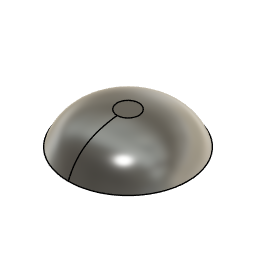
hub (Autodesk Fusion 360 archive; units mm, degrees)
design "daszek2"
Autodesk Fusion 360 part; units mm, degrees
sketch "Sketch1" plane through (0, 0, 0) normal (1, 0, 0) x (0, 1, 0)
  spline S0 degree 5 poles (-20, 0) (-22.7257, -0.3253) (-28.0984, -1.0502) (-35.9212, -2.3607) (-45.8716, -4.5618) (-57.453, -8.1224) (-68.0948, -12.571) (-77.709, -17.9907) (-86.2289, -24.4443) (-93.6692, -31.9182) (-100.0996, -40.3463) (-104.4963, -47.7952) (-107.3992, -53.7549) (-109.1618, -57.8911) (-110, -60) knots 0 0 0 0 0 0 0.1 0.2 0.3 0.4 0.5 0.6 0.7 0.8 0.9 1 1 1 1 1 1
  spline S1 degree 3 poles (-19.6445, -2.9789) (-34.008, -4.693) (-47.0407, -7.6194) (-58.39, -11.9827) (-67.6436, -15.5402) (-75.7205, -20.0828) (-82.5658, -25.7517) (-91.5958, -33.2299) (-98.5876, -42.6658) (-103.9793, -53.7643) (-105.1319, -56.1368) (-106.2094, -58.5851) (-107.2121, -61.108) knots 0 0 0 0 0.320426 0.320426 0.320426 0.581685 0.581685 0.581685 0.926327 0.926327 0.926327 1 1 1 1
  line L0 (0, 0) -> (0, -2.9702)
  line L1 (-110, -60) -> (-106.765, -60)
  line L2 (-20, 0) -> (0, 0)
  line L3 (-19.6445, -2.9789) -> (0, -2.9702)
  point P0 (-80, -20)
  dimension "d1" = 110
  dimension "d2" = 60
  dimension "d3" = 80
  dimension "d4" = 20
  dimension "d5" = -3
  dimension "d18" = 20
  constraint vertical L0
  constraint coincident S1 L1.end
  constraint perpendicular L0 L1
  constraint coincident L0.start L2.end
  constraint perpendicular L0 L2
  measures "d1" distance of L0.start S0.end
  measures "d2" distance of L0.start S0.end
  measures "d3" horizontal distance of L0.start P0
  measures "d4" vertical distance of L0.start P0
  measures "d18" distance of L0.start S0.start
revolve "Revolve1" add sketch "Sketch1" angle 360 about axis through (0, 0, 1.75) along (0, 0, 1)
ref_plane "WorkPlane1" through (0, 0, -2) normal (0, 0, 1) x (1, 0, 0)
sketch "Sketch2" plane through (0, 0, -2) normal (0, 0, 1) x (1, 0, 0)
  circle A0 centre (0, 0) radius 22.5
  dimension "d7" = 45
  constraint coincident A0.centre origin
  measures "d7" diameter of A0
extrude "Extrude1" add sketch "Sketch2" against normal blind 25
sketch "Sketch3" plane through (0, 0, -27) normal (0, 0, -1) x (1, 0, 0)
  circle A0 centre (0, 0) radius 22.5
  circle A1 centre (10.6066, -10.6066) radius 2.05
  circle A2 centre (3.8823, 14.4889) radius 2.05
  circle A3 centre (-14.4889, -3.8823) radius 2.05
  line L0 (0, 0) -> (10.6066, -10.6066) construction
  dimension "d10" = 4.1
  dimension "d14" = 360
  dimension "d19" = 15
  constraint coincident A0.centre L0.start
  constraint coincident A1.centre L0.end
  measures "d10" diameter of A1
  measures "d19" distance of A0.centre A1.centre
extrude "Extrude2" cut sketch "Sketch3" against normal blind 15 contours A1 | A2 | A3
sketch "Sketch4" plane through (0, 0, -27) normal (0, 0, -1) x (1, 0, 0)
  circle A0 centre (10.6066, -10.6066) radius 2.05
  circle A1 centre (-14.4889, -3.8823) radius 2.05
  circle A2 centre (3.8823, 14.4889) radius 2.05
  circle A3 centre (0, 0) radius 22.5
  circle A4 centre (0, 0) radius 5
  dimension "d20" = 10
  constraint concentric A3 A4
  measures "d20" diameter of A4
extrude "Extrude3" cut sketch "Sketch4" against normal blind 5 contours A4

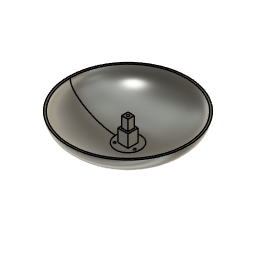
design "daszek1"
Autodesk Fusion 360 part; units mm, degrees
sketch "Sketch4" plane through (0, 0, 0) normal (0, 1, 0) x (1, 0, 0)
  spline S0 degree 5 poles (-20, 0) (-21.6536, 0) (-25.032, -0.1163) (-30.3134, -0.6396) (-37.7509, -2.0184) (-47.5071, -4.7949) (-57.4279, -8.5303) (-67.1391, -13.1315) (-76.1973, -18.5102) (-84.096, -24.5687) (-90.2992, -31.2112) (-93.4994, -36.932) (-94.7271, -41.4301) (-95, -44.5189) (-95, -46.0858) knots 0 0 0 0 0 0 0.1 0.2 0.3 0.4 0.5 0.6 0.7 0.8 0.9 1 1 1 1 1 1
  line L0 (-10, 0) -> (-30, 0)
  line L1 (-95, -36.0858) -> (-95, -56.0858)
  line L2 (-20, 0) -> (0, 0)
  line L3 (0, 0) -> (0, -3)
  spline S1 degree 3 poles (-20, -3) (-25.5966, -3) (-31.8408, -3.86) (-38.4727, -5.5163) (-46.4841, -7.517) (-55.0516, -10.6655) (-63.0384, -14.6677) (-71.1871, -18.751) (-78.7025, -23.7427) (-83.9452, -29.1422) (-87.2771, -32.5738) (-89.6623, -36.1401) (-90.918, -39.7495) (-91.6382, -41.8195) (-92, -43.9101) (-92, -46.0858) knots 0 0 0 0 0.213996 0.213996 0.213996 0.472505 0.472505 0.472505 0.736252 0.736252 0.736252 0.903871 0.903871 0.903871 1 1 1 1
  line L4 (-20, -3) -> (0, -3)
  line L5 (-95, -46.0858) -> (-92, -46.0858)
  point P0 (-70, -15)
  dimension "d30" = 20
  dimension "d45" = 3
  dimension "d46" = -3
  constraint coincident L2.end L3.start
  constraint perpendicular L2 L3
  measures "d30" distance of S0.start L2.end
  measures "d45" distance of L2.end L3.end
revolve "Revolve1" add sketch "Sketch4" angle 360 about axis through (0, 0, 1.75) along (0, 0, 1) makes body 1
sketch "Sketch5" plane through (0, 0, 3) normal (0, 0, 1) x (-1, 0, 0)
  line L0 (5, 5) -> (-5, 5)
  line L1 (-5, 5) -> (-5, -5)
  line L2 (-5, -5) -> (5, -5)
  line L3 (5, -5) -> (5, 5)
  line L4 (5, 5) -> (-5, -5) construction
  line L5 (-5, 5) -> (5, -5) construction
  line L6 (-8, 8) -> (-8, -8)
  line L7 (-8, -8) -> (8, -8)
  line L8 (8, -8) -> (8, 8)
  line L9 (8, 8) -> (-8, 8)
  circle A0 centre (0, 0) radius 20
  dimension "d33" = 10
  dimension "d34" = 10
  dimension "d35" = 3
  constraint horizontal L0
  constraint perpendicular L0 L1
  constraint parallel L0 L2
  constraint parallel L1 L3
  constraint coincident L4 A0.centre
  constraint coincident L5 A0.centre
  measures "d33" distance of L1.end L2.end
  measures "d34" distance of L0.end L1.end
extrude "Extrude2" add sketch "Sketch5" along normal blind 37 separate body contours L0 L1 L2 L3 makes body 2
sketch "Sketch6" plane through (0, 0, 40) normal (0, 0, 1) x (-1, 0, 0)
  circle A0 centre (0, 0) radius 2.05
  line L0 (5, -5) -> (5, 5)
  line L1 (5, 5) -> (-5, 5)
  line L2 (-5, 5) -> (-5, -5)
  line L3 (-5, -5) -> (5, -5)
  dimension "d16" = 4.1
  constraint coincident A0.centre origin
  measures "d16" diameter of A0
extrude "Extrude3" cut sketch "Sketch6" against normal blind 15 contours A0 bodies 2 1
sketch "Sketch7" plane through (0, 0, 0) normal (0, 0, -1) x (1, 0, 0)
  circle A0 centre (0, 0) radius 20
  circle A1 centre (-10.6066, 10.6066) radius 1.75
  circle A2 centre (-3.8823, -14.4889) radius 1.75
  circle A3 centre (14.4889, 3.8823) radius 1.75
  line L0 (0, 0) -> (-10.6066, 10.6066) construction
  dimension "d19" = 3.5
  dimension "d23" = 360
  dimension "d32" = 15
  constraint coincident A0.centre L0.start
  constraint coincident A1.centre L0.end
  measures "d19" diameter of A1
  measures "d32" distance of A0.centre A1.centre
extrude "Extrude4" cut sketch "Sketch7" against normal blind 15 contours A1 | A2 | A3 bodies 1 2
extrude "Extrude7" add sketch "Sketch5" along normal blind 20 contours L6 L7 L8 L9 bodies 1
sketch "Sketch9" plane through (0, 0, 3) normal (0, 0, 1) x (-1, 0, 0)
  line L0 (5, 5) -> (-5, 5)
  line L1 (-5, 5) -> (-5, -5)
  line L2 (-5, -5) -> (5, -5)
  line L3 (5, -5) -> (5, 5)
  circle A0 centre (0, 0) radius 1.75
  circle A1 centre (0, 0) radius 20
  circle A2 centre (3.8823, -14.4889) radius 1.75
  circle A3 centre (-14.4889, 3.8823) radius 1.75
  circle A4 centre (10.6066, 10.6066) radius 1.75
  line L4 (8, 8) -> (8, -8)
  line L5 (8, -8) -> (-8, -8)
  line L6 (-8, -8) -> (-8, 8)
  line L7 (-8, 8) -> (8, 8)
  dimension "d39" = 3.5
  constraint coincident A0.centre A1.centre
  measures "d39" diameter of A0
extrude "Extrude8" cut sketch "Sketch9" against normal blind 5 contours A0 bodies 1
extrude "Extrude9" cut sketch "Sketch9" along normal blind 10 contours A0 bodies 2

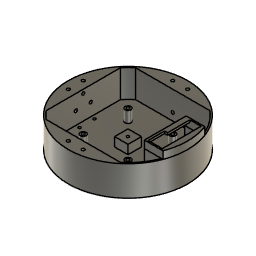
design "obudowa"
Autodesk Fusion 360 part; units mm, degrees
sketch "Sketch1" plane through (0, 0, 0) normal (0, 0, 1) x (1, 0, 0)
  circle A0 centre (0, 0) radius 80
  circle A1 centre (0, 0) radius 78
  dimension "d1" = 160
  dimension "d2" = -2
  constraint coincident A0.centre A1.centre
  measures "d1" diameter of A0
extrude "Extrude1" add sketch "Sketch1" along normal blind 3 contours A1 makes body 1
extrude "Extrude2" add sketch "Sketch1" along normal blind 40 bodies 1
sketch "Sketch2" plane through (0, 0, 3) normal (0, 0, 1) x (-1, 0, 0)
  circle A0 centre (0, 0) radius 78
  circle A1 centre (30, -30) radius 2.05
  circle A2 centre (30, -30) radius 4
  circle A3 centre (30, 30) radius 2.05
  circle A4 centre (30, 30) radius 4
  circle A5 centre (-30, 30) radius 2.05
  circle A6 centre (-30, 30) radius 4
  circle A7 centre (-30, -30) radius 2.05
  circle A8 centre (-30, -30) radius 4
  dimension "d7" = 4.1
  dimension "d8" = 8
  dimension "d9" = 30
  dimension "d10" = 30
  dimension "d12" = 360
  constraint concentric A1 A2
  measures "d7" diameter of A1
  measures "d8" diameter of A2
  measures "d9" horizontal distance of A0.centre A1.centre
  measures "d10" vertical distance of A0.centre A1.centre
extrude "Extrude3" add sketch "Sketch2" along normal blind 15 contours A2 | A4 | A6 | A8 bodies 1
sketch "Sketch14" plane through (0, 0, 3) normal (0, 0, 1) x (-1, 0, 0)
  circle A0 centre (30, -30) radius 4
  circle A1 centre (-30, -30) radius 4
  circle A2 centre (0, 0) radius 78
  circle A3 centre (-30, 30) radius 4
  circle A4 centre (30, 30) radius 4
sketch "Sketch15" plane through (0, 0, 3) normal (0, 0, 1) x (-1, 0, 0)
  line L0 (-50, 28) -> (-50, -28)
  line L1 (-72.8011, 28) -> (-46, 28)
  line L2 (-72.8011, -28) -> (-41.8968, -28)
  circle A0 centre (0, 0) radius 78
  line L3 (-73.5391, 26) -> (-46, 26)
  line L4 (-73.5391, -26) -> (-46, -26)
  dimension "d80" = 50
  dimension "d81" = 28
  dimension "d82" = 28
  dimension "d83" = 2
  dimension "d84" = 2
  constraint vertical L0
  constraint perpendicular L0 L1
  constraint horizontal L2
  constraint coincident L1.start A0
  constraint coincident L2.start A0
  constraint coincident L0.start L1
  constraint coincident L0.end L2
  constraint coincident A0 L3.start
  constraint parallel L1 L3
  constraint coincident A0 L4.start
  constraint perpendicular L0 L4
  measures "d80" distance of L0 A0.centre
  measures "d81" distance of A0.centre L1
  measures "d82" distance of L2 A0.centre
  measures "d83" distance of L2 L4
  measures "d84" distance of L1 L3
extrude "Extrude5" add sketch "Sketch15" along normal blind 37 contours L0 L1 A0 L3 | L0 L2 A0 L4 bodies 1
sketch "Sketch4" plane through (0, -28, 0) normal (0, -1, 0) x (1, 0, 0)
  line L0 (50.5391, 3) -> (72.8011, 3)
  line L1 (72.8011, 3) -> (72.8011, 40)
  line L2 (72.8011, 40) -> (50.5391, 40)
  line L3 (50.5391, 40) -> (50.5391, 3)
  circle A0 centre (55.5391, 20) radius 2
  line L4 (50, 3) -> (72.8011, 3)
  line L5 (72.8011, 3) -> (72.8011, 40)
  line L6 (72.8011, 40) -> (50, 40)
  line L7 (50, 40) -> (50, 3)
  dimension "d25" = 4
  dimension "d26" = 5
  dimension "d27" = 20
  measures "d25" diameter of A0
  measures "d26" distance of L3 A0.centre
  measures "d27" distance of L2 A0.centre
ref_plane "WorkPlane1" through (55.5391, -34, 20) normal (0, -1, 0) x (1, 0, 0)
sketch "Sketch5" plane through (55.5391, -34, 20) normal (0, -1, 0) x (1, 0, 0)
  circle A0 centre (0, 0) radius 1.25
  dimension "d29" = 2.5
  constraint coincident A0.centre origin
  measures "d29" diameter of A0
loft "Loft1" add profiles "Sketch4", "Sketch5" section 1 contours A0 section 2 bodies 1
sketch "Sketch6" plane through (0, 0, 3) normal (0, 0, 1) x (-1, 0, 0)
  circle A0 centre (30, 30) radius 4
  circle A1 centre (-30, 30) radius 4
  circle A2 centre (-30, -30) radius 4
  circle A3 centre (30, -30) radius 4
  arc A4 (-72.8011, -28) -> (-72.8011, 28) centre (0, 0) ccw
  line L0 (-50, -28) -> (-72.8011, -28)
  line L1 (-72.8011, 28) -> (-50, 28)
  line L2 (-50, 28) -> (-50, 26)
  line L3 (-50, 26) -> (-73.5391, 26)
  arc A5 (-73.5391, 26) -> (-73.5391, -26) centre (0, 0) ccw
  line L4 (-73.5391, -26) -> (-50, -26)
  line L5 (-50, -26) -> (-50, -28)
  line L6 (-5, -5) -> (5, -5)
  line L7 (5, -5) -> (5, 5)
  line L8 (5, 5) -> (-5, 5)
  line L9 (-5, 5) -> (-5, -5)
  line L10 (-5, -5) -> (5, 5) construction
  line L11 (5, -5) -> (-5, 5) construction
  line L12 (-9, -9) -> (9, -9)
  line L13 (9, -9) -> (9, 9)
  line L14 (9, 9) -> (-9, 9)
  line L15 (-9, 9) -> (-9, -9)
  line L16 (-9, -9) -> (9, 9) construction
  line L17 (9, -9) -> (-9, 9) construction
  dimension "d100" = 10
  dimension "d101" = 10
  dimension "d102" = 18
  dimension "d103" = 18
  constraint horizontal L6
  constraint perpendicular L6 L7
  constraint parallel L6 L8
  constraint parallel L7 L9
  constraint coincident L10 A4.centre
  constraint coincident L11 A4.centre
  constraint coincident A4.centre A5.centre
  constraint horizontal L12
  constraint perpendicular L12 L13
  constraint parallel L12 L14
  constraint parallel L13 L15
  constraint coincident L16 A4.centre
  constraint coincident L17 A4.centre
  measures "d100" distance of L7.end L8.end
  measures "d101" distance of L6.end L7.end
  measures "d102" distance of L13.end L14.end
  measures "d103" distance of L12.end L13.end
extrude "Extrude7" cut sketch "Sketch6" against normal blind 3 contours L6 L7 L8 L9 bodies 1
extrude "Extrude18" add sketch "Sketch6" along normal blind 12 contours L6 L7 L8 L9 | L12 L13 L14 L15 bodies 1
extrude "Extrude20" cut 1 faces at (1.6667, -1.6667, 3) along direction (0, 0, 1) blind 7 on bodies 1 bodies 1
sketch "Sketch19" plane through (0, 0, 15) normal (0, 0, 1) x (-1, 0, 0)
  circle A0 centre (0, 0) radius 1.75
  line L0 (-9, 9) -> (-9, -9)
  line L1 (-9, -9) -> (9, -9)
  line L2 (9, -9) -> (9, 9)
  line L3 (9, 9) -> (-9, 9)
  dimension "d97" = 3.5
  constraint coincident A0.centre origin
  measures "d97" diameter of A0
extrude "Extrude19" cut sketch "Sketch19" against normal blind 5 contours A0 bodies 1
sketch "Sketch7" plane through (0, 0, 40) normal (0, 0, 1) x (-1, 0, 0)
  arc A0 (-72.8011, -28) -> (-72.8011, 28) centre (0, 0) ccw
  circle A1 centre (0, 0) radius 80
  line L0 (60, 49.8397) -> (60, -49.8397)
  line L1 (-72.8011, -28) -> (-50, -28)
  line L2 (-50, -28) -> (-50, -26)
  line L3 (-50, -26) -> (-73.5391, -26)
  arc A2 (-73.5391, 26) -> (-73.5391, -26) centre (0, 0) ccw
  line L4 (-73.5391, 26) -> (-50, 26)
  line L5 (-50, 26) -> (-50, 28)
  line L6 (-50, 28) -> (-72.8011, 28)
  dimension "d33" = 60
  constraint vertical L0
  constraint coincident A0 L0.start
  constraint coincident A0 L0.end
  measures "d33" distance of A0.centre L0
extrude "Extrude8" add sketch "Sketch7" against normal blind 37 contours A0 L0 bodies 1
sketch "Sketch8" plane through (0, 0, 3) normal (0, 0, 1) x (-1, 0, 0)
  line L0 (60, -49.8397) -> (60, 49.8397)
  arc A0 (60, 49.8397) -> (-72.8011, 28) centre (0, 0) ccw
  circle A1 centre (30, 30) radius 4
  circle A2 centre (-30, 30) radius 4
  circle A3 centre (-30, -30) radius 4
  circle A4 centre (30, -30) radius 4
  circle A5 centre (55, -10) radius 1.75
  line L1 (10, 0) -> (18.1921, 0) construction
  circle A6 centre (55, 10) radius 1.75
  line L2 (-72.8011, 28) -> (-50, 28)
  line L3 (-50, 28) -> (-50, 26)
  line L4 (-50, 26) -> (-73.5391, 26)
  arc A7 (-73.5391, 26) -> (-73.5391, -26) centre (0, 0) ccw
  line L5 (-73.5391, -26) -> (-50, -26)
  line L6 (-50, -26) -> (-50, -28)
  line L7 (-50, -28) -> (-72.8011, -28)
  arc A8 (-72.8011, -28) -> (60, -49.8397) centre (0, 0) ccw
  line L8 (-9, 9) -> (9, 9)
  line L9 (9, 9) -> (9, -9)
  line L10 (9, -9) -> (-9, -9)
  line L11 (-9, -9) -> (-9, 9)
  dimension "d36" = 3.5
  dimension "d37" = 5
  dimension "d38" = 10
  constraint horizontal L1
  constraint symmetric A5 L1 A6
  constraint horizontal A0.centre L1.start
  measures "d36" diameter of A5
  measures "d37" distance of L0 A5.centre
  measures "d38" vertical distance of A0.centre A5.centre
extrude "Extrude9" cut sketch "Sketch8" against normal blind 3 contours A5 | A6 bodies 1
sketch "Sketch9" plane through (-60, 0, 0) normal (1, 0, 0) x (0, 1, 0)
  line L0 (49.8397, 40) -> (-49.8397, 40)
  line L1 (-49.8397, 40) -> (-49.8397, 3)
  line L2 (-49.8397, 3) -> (49.8397, 3)
  line L3 (49.8397, 3) -> (49.8397, 40)
  circle A0 centre (-10, 20) radius 2.05
  circle A1 centre (10, 20) radius 2.05
  circle A2 centre (0, 35) radius 2.05
  line L4 (0, 0) -> (0, 13)
  dimension "d41" = 4.1
  dimension "d42" = 4.1
  dimension "d43" = 10
  dimension "d44" = 10
  dimension "d45" = 20
  dimension "d46" = 20
  dimension "d47" = 4.1
  dimension "d48" = 35
  constraint coincident L4.start origin
  constraint perpendicular L2 L4
  constraint coincident A2.centre L4
  measures "d41" diameter of A0
  measures "d42" diameter of A1
  measures "d43" horizontal distance of L4.start A1.centre
  measures "d44" horizontal distance of L4.start A0.centre
  measures "d45" vertical distance of L4.start A1.centre
  measures "d46" vertical distance of L4.start A0.centre
  measures "d47" diameter of A2
  measures "d48" distance of L4.start A2.centre
extrude "Extrude10" cut sketch "Sketch9" against normal blind 8 contours A0 | A1 | A2 bodies 1
sketch "Sketch10" plane through (0, 0, 40) normal (0, 0, 1) x (-1, 0, 0)
  arc A0 (60, 49.8397) -> (-72.8011, 28) centre (0, 0) ccw
  line L0 (60, 49.8397) -> (60, -49.8397)
  arc A1 (-72.8011, -28) -> (60, -49.8397) centre (0, 0) ccw
  circle A2 centre (0, 0) radius 80
  circle A3 centre (70, -10) radius 2.05
  circle A4 centre (70, 10) radius 2.05
  line L1 (-72.8011, -28) -> (-50, -28)
  line L2 (-50, -28) -> (-50, -26)
  line L3 (-50, -26) -> (-73.5391, -26)
  arc A5 (-73.5391, 26) -> (-73.5391, -26) centre (0, 0) ccw
  line L4 (-73.5391, 26) -> (-50, 26)
  line L5 (-50, 26) -> (-50, 28)
  line L6 (-50, 28) -> (-72.8011, 28)
  dimension "d51" = 4.1
  dimension "d52" = 4.1
  dimension "d53" = 10
  dimension "d54" = 10
  dimension "d55" = 10
  dimension "d56" = 10
  measures "d51" diameter of A3
  measures "d52" diameter of A4
  measures "d53" vertical distance of A0.centre A4.centre
  measures "d54" vertical distance of A0.centre A3.centre
  measures "d55" distance of L0 A3.centre
  measures "d56" distance of L0 A4.centre
extrude "Extrude11" cut sketch "Sketch10" against normal blind 8 contours A3 | A4 bodies 1
sketch "Sketch11" plane through (0, 0, 40) normal (0, 0, 1) x (-1, 0, 0)
  circle A0 centre (70, -10) radius 2.05
  circle A1 centre (70, 10) radius 2.05
  arc A2 (60, 49.8397) -> (-72.8011, 28) centre (0, 0) ccw
  line L0 (60, 49.8397) -> (60, -49.8397)
  arc A3 (-72.8011, -28) -> (60, -49.8397) centre (0, 0) ccw
  circle A4 centre (0, 0) radius 80
  line L1 (49.8397, -60) -> (-49.8397, -60)
  line L2 (-72.8011, -28) -> (-50, -28)
  line L3 (-50, -28) -> (-50, -26)
  line L4 (-50, -26) -> (-73.5391, -26)
  arc A5 (-73.5391, 26) -> (-73.5391, -26) centre (0, 0) ccw
  line L5 (-73.5391, 26) -> (-50, 26)
  line L6 (-50, 26) -> (-50, 28)
  line L7 (-50, 28) -> (-72.8011, 28)
  dimension "d59" = 60
  constraint horizontal L1
  constraint coincident A3 L1.start
  constraint coincident A3 L1.end
  measures "d59" distance of A2.centre L1
extrude "Extrude12" add sketch "Sketch11" against normal blind 37 contours A3 L1 bodies 1
sketch "Sketch12" plane through (0, 60, 0) normal (0, -1, 0) x (1, 0, 0)
  line L0 (49.8397, 40) -> (-49.8397, 40)
  line L1 (-49.8397, 40) -> (-49.8397, 3)
  line L2 (-49.8397, 3) -> (49.8397, 3)
  line L3 (49.8397, 3) -> (49.8397, 40)
  circle A0 centre (0, 13) radius 2.05
  dimension "d62" = 4.1
  dimension "d63" = 10
  constraint vertical origin A0.centre
  measures "d62" diameter of A0
  measures "d63" distance of L2 A0.centre
extrude "Extrude13" cut sketch "Sketch12" against normal blind 8 contours A0 bodies 1
sketch "Sketch13" plane through (0, 0, 40) normal (0, 0, 1) x (-1, 0, 0)
  circle A0 centre (70, -10) radius 2.05
  circle A1 centre (70, 10) radius 2.05
  arc A2 (60, 49.8397) -> (-72.8011, 28) centre (0, 0) ccw
  line L0 (60, 49.8397) -> (60, -49.8397)
  arc A3 (49.8397, -60) -> (60, -49.8397) centre (0, 0) ccw
  line L1 (49.8397, -60) -> (-49.8397, -60)
  arc A4 (-72.8011, -28) -> (-49.8397, -60) centre (0, 0) ccw
  circle A5 centre (0, 0) radius 80
  circle A6 centre (10, -70) radius 2.05
  circle A7 centre (-10, -70) radius 2.05
  line L2 (-72.8011, -28) -> (-50, -28)
  line L3 (-50, -28) -> (-50, -26)
  line L4 (-50, -26) -> (-73.5391, -26)
  arc A8 (-73.5391, 26) -> (-73.5391, -26) centre (0, 0) ccw
  line L5 (-73.5391, 26) -> (-50, 26)
  line L6 (-50, 26) -> (-50, 28)
  line L7 (-50, 28) -> (-72.8011, 28)
  dimension "d66" = 4.1
  dimension "d67" = 4.1
  dimension "d68" = 10
  dimension "d69" = 10
  dimension "d70" = 10
  dimension "d71" = 10
  measures "d66" diameter of A6
  measures "d67" diameter of A7
  measures "d68" distance of L1 A6.centre
  measures "d69" distance of L1 A7.centre
  measures "d70" horizontal distance of A2.centre A6.centre
  measures "d71" horizontal distance of A2.centre A7.centre
extrude "Extrude14" cut sketch "Sketch13" against normal blind 8 contours A6 | A7 bodies 1
mirror "Mirror1" about plane through (0, 0, 0) normal (0, 1, 0) of "Extrude12", "Extrude13", "Extrude14"
sketch "Sketch16" plane through (0, 0, 3) normal (0, 0, 1) x (-1, 0, 0)
  line L0 (-72, 26) -> (-72, -26)
  circle A0 centre (0, 0) radius 78
  line L1 (-50, 26) -> (-73.5391, 26)
  line L2 (-73.5391, -26) -> (-50, -26)
  dimension "d86" = 72
  constraint vertical L0
  measures "d86" distance of L0 A0.centre
extrude "Extrude15" add sketch "Sketch16" along normal blind 37 separate body contours L0 A0 L1 L2 picked at (-73.4614, -5.2648) makes body 2
sketch "Sketch17" plane through (0, 0, 40) normal (0, 0, 1) x (-1, 0, 0)
  line L0 (-72, 26) -> (-73.5391, 26)
  arc A0 (-73.5391, 26) -> (-73.5391, -26) centre (0, 0) ccw
  line L1 (-73.5391, -26) -> (-72, -26)
  line L2 (-72, -26) -> (-72, 26)
  circle A1 centre (10, 70) radius 2.05
  circle A2 centre (-10, 70) radius 2.05
  circle A3 centre (10, -70) radius 2.05
  circle A4 centre (-10, -70) radius 2.05
  circle A5 centre (70, -10) radius 2.05
  circle A6 centre (70, 10) radius 2.05
  arc A7 (-49.8397, 60) -> (-72.8011, 28) centre (0, 0) ccw
  line L3 (-49.8397, 60) -> (49.8397, 60)
  arc A8 (60, 49.8397) -> (49.8397, 60) centre (0, 0) ccw
  line L4 (60, 49.8397) -> (60, -49.8397)
  arc A9 (49.8397, -60) -> (60, -49.8397) centre (0, 0) ccw
  line L5 (49.8397, -60) -> (-49.8397, -60)
  arc A10 (-72.8011, -28) -> (-49.8397, -60) centre (0, 0) ccw
  line L6 (-72.8011, -28) -> (-50, -28)
  line L7 (-50, -28) -> (-50, -26)
  line L8 (-50, -26) -> (-73.5391, -26)
  arc A11 (-73.5391, 26) -> (-73.5391, -26) centre (0, 0) ccw
  line L9 (-73.5391, 26) -> (-50, 26)
  line L10 (-50, 26) -> (-50, 28)
  line L11 (-50, 28) -> (-72.8011, 28)
  circle A12 centre (0, 0) radius 80
  line L12 (-72.8011, -28) -> (-74.94, -28)
  line L13 (-72.8011, 28) -> (-74.94, 28)
  constraint coincident A10.start L6.start
  constraint coincident A12 L12.end
  constraint parallel L6 L12
  constraint coincident A7.end L11.end
  constraint coincident A12 L13.end
  constraint parallel L11 L13
extrude "Extrude16" add sketch "Sketch17" along normal blind 10 separate body contours L0 A0 L1 L2 L8 A11 L9 | L0 A0 L1 L6 L7 L8 A11 L9 L10 L11 A12 L12 L13 makes body 3
sketch "Sketch18" plane through (0, 0, 50) normal (0, 0, 1) x (-1, 0, 0)
  line L0 (-74.94, -28) -> (-50, -28)
  line L1 (-50, -28) -> (-50, -26)
  line L2 (-50, -26) -> (-72, -26)
  line L3 (-72, -26) -> (-72, 26)
  line L4 (-72, 26) -> (-50, 26)
  line L5 (-50, 26) -> (-50, 28)
  line L6 (-50, 28) -> (-74.94, 28)
  arc A0 (-74.94, 28) -> (-74.94, -28) centre (0, 0) ccw
  line L7 (-72, -26) -> (-50, -26)
  line L8 (-50, -26) -> (-50, 4)
  line L9 (-50, 4) -> (-72, 4)
  line L10 (-72, 4) -> (-72, -26)
  line L11 (-50, 26) -> (-53, 26)
  line L12 (-53, 26) -> (-53, 4)
  line L13 (-53, 4) -> (-50, 4)
  line L14 (-50, 4) -> (-50, 26)
  line L15 (-72, 4) -> (-57, 4)
  line L16 (-57, 4) -> (-57, -26)
  line L17 (-57, -26) -> (-72, -26)
  line L18 (-72, -26) -> (-72, 4)
  dimension "d106" = 15
  constraint horizontal L7
  constraint vertical L8
  constraint horizontal L9
  constraint vertical L10
  constraint coincident L2.end L3.start
  constraint horizontal L11
  constraint vertical L12
  constraint horizontal L13
  constraint vertical L14
  constraint coincident L9 L12.end
  constraint coincident L4.end L5.start
  constraint horizontal L15
  constraint vertical L16
  constraint horizontal L17
  constraint vertical L18
  measures "d106" distance of L9.end L15.end
extrude "Extrude17" add sketch "Sketch18" against normal blind 3 contours L2 L7 L8 L9 L13 L16 | L4 L9 L11 L12 L13 L14 bodies 3
combine "Combine1" operation add target body 3 tool bodies 2

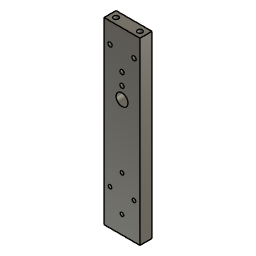
design "mocowanie"
Autodesk Fusion 360 part; units mm, degrees
sketch "Sketch1" plane through (0, 0, 0) normal (0, 0, 1) x (1, 0, 0)
  line L0 (15, 5) -> (-15, 5)
  line L1 (-15, 5) -> (-15, -5)
  line L2 (-15, -5) -> (15, -5)
  line L3 (15, -5) -> (15, 5)
  line L4 (15, 5) -> (-15, -5) construction
  line L5 (-15, 5) -> (15, -5) construction
  dimension "d1" = 30
  dimension "d2" = 10
  constraint horizontal L0
  constraint perpendicular L0 L1
  constraint parallel L0 L2
  constraint parallel L1 L3
  constraint coincident L4 origin
  constraint coincident L5 origin
  measures "d1" distance of L1.end L2.end
  measures "d2" distance of L0.end L1.end
extrude "Extrude1" add sketch "Sketch1" along normal blind 150
sketch "Sketch2" plane through (0, -5, 0) normal (0, -1, 0) x (1, 0, 0)
  line L0 (-15, 0) -> (15, 0)
  line L1 (15, 0) -> (15, 150)
  line L2 (15, 150) -> (-15, 150)
  line L3 (-15, 150) -> (-15, 0)
  circle A0 centre (0, 118) radius 1.75
  line L4 (0, 150) -> (0, 118)
  circle A1 centre (-10, 133) radius 1.75
  circle A2 centre (10, 133) radius 1.75
  dimension "d5" = 3.5
  dimension "d6" = 32
  dimension "d7" = 3.5
  dimension "d8" = 3.5
  dimension "d9" = 10
  dimension "d10" = 10
  dimension "d11" = 15
  dimension "d12" = 15
  constraint midpoint L2 L4.start
  constraint perpendicular L2 L4
  constraint coincident A0.centre L4.end
  measures "d5" diameter of A0
  measures "d6" distance of L2 A0.centre
  measures "d7" diameter of A1
  measures "d8" diameter of A2
  measures "d9" distance of L4 A1.centre
  measures "d10" distance of L4 A2.centre
  measures "d11" vertical distance of A0.centre A1.centre
  measures "d12" vertical distance of A0.centre A2.centre
extrude "Extrude2" cut sketch "Sketch2" against normal blind 10 contours A0 | A1 | A2
sketch "Sketch3" plane through (0, 0, 150) normal (0, 0, 1) x (-1, 0, 0)
  line L0 (-15, 5) -> (-15, -5)
  line L1 (-15, -5) -> (15, -5)
  line L2 (15, -5) -> (15, 5)
  line L3 (15, 5) -> (-15, 5)
  circle A0 centre (10, 0) radius 2.05
  circle A1 centre (-10, 0) radius 2.05
  dimension "d15" = 4.1
  dimension "d17" = 10
  dimension "d18" = 10
  constraint equal A0 A1
  constraint horizontal origin A0.centre
  constraint horizontal origin A1.centre
  measures "d15" diameter of A0
  measures "d17" distance of origin A0.centre
  measures "d18" distance of origin A1.centre
extrude "Extrude3" cut sketch "Sketch3" against normal blind 12 contours A0 | A1
sketch "Sketch4" plane through (0, -5, 0) normal (0, -1, 0) x (1, 0, 0)
  circle A0 centre (-10, 133) radius 1.75
  circle A1 centre (10, 133) radius 1.75
  circle A2 centre (0, 118) radius 1.75
  line L0 (-15, 0) -> (15, 0)
  line L1 (15, 0) -> (15, 150)
  line L2 (15, 150) -> (-15, 150)
  line L3 (-15, 150) -> (-15, 0)
  line L4 (0, 0) -> (0, 6)
  circle A3 centre (0, 15) radius 1.5
  circle A4 centre (-10, 30) radius 1.5
  circle A5 centre (10, 30) radius 1.5
  circle A6 centre (0, 45) radius 1.5
  dimension "d21" = 3
  dimension "d22" = 15
  dimension "d23" = 3
  dimension "d24" = 10
  dimension "d25" = 30
  dimension "d26" = 3
  dimension "d27" = 45
  constraint coincident L4.start origin
  constraint perpendicular L0 L4
  constraint coincident L4 A3.centre
  constraint symmetric L4 A4 A5
  constraint coincident L4 A6.centre
  measures "d21" diameter of A3
  measures "d22" distance of L0 A3.centre
  measures "d23" diameter of A4
  measures "d24" horizontal distance of L4.start A4.centre
  measures "d25" vertical distance of L4.start A4.centre
  measures "d26" diameter of A6
  measures "d27" distance of L0 A6.centre
extrude "Extrude4" cut sketch "Sketch4" against normal blind 10 contours A3 | A4 | A5 | A6
sketch "Sketch5" plane through (0, -5, 0) normal (0, -1, 0) x (1, 0, 0)
  circle A0 centre (0, 45) radius 1.5
  circle A1 centre (10, 30) radius 1.5
  circle A2 centre (-10, 30) radius 1.5
  circle A3 centre (0, 15) radius 1.5
  circle A4 centre (-10, 133) radius 1.75
  circle A5 centre (10, 133) radius 1.75
  circle A6 centre (0, 118) radius 1.75
  line L0 (-15, 0) -> (15, 0)
  line L1 (15, 0) -> (15, 150)
  line L2 (15, 150) -> (-15, 150)
  line L3 (-15, 150) -> (-15, 0)
  circle A7 centre (0, 108) radius 1.75
  dimension "d30" = 3.5
  dimension "d31" = 10
  measures "d30" diameter of A7
  measures "d31" distance of A6.centre A7.centre
extrude "Extrude5" cut sketch "Sketch5" against normal blind 10 contours A7
sketch "Sketch6" plane through (0, -5, 0) normal (0, -1, 0) x (1, 0, 0)
  circle A0 centre (0, 108) radius 1.75
  circle A1 centre (0, 45) radius 1.5
  circle A2 centre (10, 30) radius 1.5
  circle A3 centre (-10, 30) radius 1.5
  circle A4 centre (0, 15) radius 1.5
  circle A5 centre (-10, 133) radius 1.75
  circle A6 centre (10, 133) radius 1.75
  circle A7 centre (0, 118) radius 1.75
  line L0 (-15, 0) -> (15, 0)
  line L1 (15, 0) -> (15, 150)
  line L2 (15, 150) -> (-15, 150)
  line L3 (-15, 150) -> (-15, 0)
  circle A8 centre (0, 98) radius 5
  dimension "d34" = 10
  dimension "d35" = 10
  measures "d34" diameter of A8
  measures "d35" distance of A0.centre A8.centre
extrude "Extrude6" cut sketch "Sketch6" against normal blind 10 contours A8
